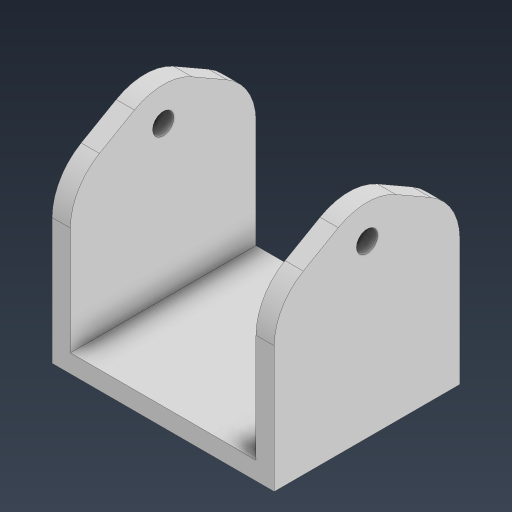
# Autodesk Inventor part: Cover
Saved by Autodesk Inventor 2024 (Build 280153000, 153)
## iProperties
Created: 2023-12-28
Part Number: Cover
Material: Generic
Document SubType Name: Modeling
Designer: Piter
Density: 1 g/cm^3
Appearance: Default
Author: Piter
Autodesk Inventor part; units mm, degrees
ref_plane "YZ Plane" through (0, 0, 0) normal (1, 0, 0) x (0, 1, 0)
ref_plane "XZ Plane" through (0, 0, 0) normal (0, 1, 0) x (-1, 0, 0)
ref_plane "XY Plane" through (0, 0, 0) normal (0, 0, 1) x (1, 0, 0)
sketch "Sketch1" plane through (0, 0, 0) normal (0, 1, 0) x (-1, 0, 0)
  line L0 (0, 0) -> (30.5, 0)
  line L1 (30.5, 0) -> (30.5, -30.5)
  line L2 (30.5, -30.5) -> (0, -30.5)
  line L3 (0, -30.5) -> (0, 0)
  line L4 (30.5, 0) -> (33.5, 0)
  line L5 (33.5, 0) -> (33.5, -30.5)
  line L6 (33.5, -30.5) -> (30.5, -30.5)
  line L7 (30.5, -30.5) -> (30.5, 0)
  line L8 (0, -30.5) -> (-3, -30.5)
  line L9 (-3, -30.5) -> (-3, 0)
  line L10 (-3, 0) -> (0, 0)
  line L11 (0, 0) -> (0, -30.5)
  dimension "d0" = 30.5
  dimension "d1" = 30.5
  dimension "d2" = 3
  dimension "d3" = 3
  constraints: 24 end point, 6 parallel, 3 horizontal, 3 perpendicular, 1 point on line
  measures "d0" distance of L1.end L2.end
  measures "d1" distance of L0.end L1.end
  measures "d2" distance of L5.end L6.end
  measures "d3" distance of L9.end L10.end
extrude "Extrusion1" add sketch "Sketch1" along normal blind 3 contours L0 L1 L2 L3
extrude "Extrusion2" add sketch "Sketch1" along normal blind 35 contours L3 L8 L9 L10 | L4 L5 L6 L1
sketch "Sketch2" plane through (3, 0, 0) normal (1, 0, 0) x (0, 0, -1)
  line L0 (0, 3) -> (30.5, 3) projected
  line L1 (15.25, 3) -> (15.25, 28)
  circle A0 centre (15.25, 28) radius 1.75
  line L2 (30.5, 35) -> (0, 35) projected
  line L3 (15.25, 35) -> (0, 26.25)
  line L4 (0, 3) -> (0, 35) projected
  line L5 (15.25, 35) -> (30.5, 26.25)
  line L6 (30.5, 35) -> (30.5, 26.25)
  point P0 (0, 0)
  dimension "d8" = 3.5
  dimension "d9" = 25
  constraints: 8 end point, 2 midpoint, 2 point on line, 2 vertical, 1 centre point, 1 coincident
  measures "d8" diameter of A0
  measures "d9" distance of L1.start L1.end
extrude "Extrusion3" cut sketch "Sketch2" against normal through all
fillet "Fillet1" radius 9.5 6 edges at (1.5, 35, -15.25) (-32, 35, -15.25) (-32, 26.25, -30.5) (-32, 26.25, 0) (1.5, 26.25, 0) (1.5, 26.25, -30.5)
body "Solid1"
